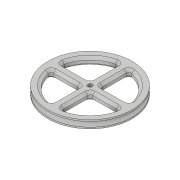
# Autodesk Inventor part: Wheel
Saved by Autodesk Inventor 2017 (Build 210142000, 142)
## iProperties
Created: 2019-06-10
Part Number: Wheel
Material: Generic
Document SubType Name: Modeling
Designer: markg
Density: 1 g/cm^3
Appearance: Default
Author: markg
Autodesk Inventor part; units mm, degrees
ref_plane "YZ Plane" through (0, 0, 0) normal (1, 0, 0) x (0, 1, 0)
ref_plane "XZ Plane" through (0, 0, 0) normal (0, 1, 0) x (-1, 0, 0)
ref_plane "XY Plane" through (0, 0, 0) normal (0, 0, 1) x (1, 0, 0)
sketch "Sketch1" plane through (0, 0, 0) normal (0, 0, 1) x (1, 0, 0)
  line L0 (0, 0) -> (26.9875, 0)
  line L1 (26.9875, 5.08) -> (0, 5.08)
  line L2 (0, 5.08) -> (0, 0)
  arc A0 (26.9875, 4.1275) -> (26.9875, 0.9525) centre (26.9875, 2.54) ccw
  line L3 (26.9875, 0) -> (26.9875, 0.9525)
  line L4 (26.9875, 4.1275) -> (26.9875, 5.08)
  dimension "d0" = 5.08
  dimension "d1" = 26.9875
  dimension "d2" = 3.175
  constraints: 10 end point, 3 parallel, 2 perpendicular, 2 point on circle, 1 centre point, 1 horizontal
  measures "d0" distance of L0.end L1.start
  measures "d1" distance of L1.start L1.end
  measures "d2" diameter of A0
revolve "Revolution1" add sketch "Sketch1" angle 360 about axis through (0, 5.08, 0) along (0, -1, 0)
sketch "Sketch2" plane through (0, 5.08, 0) normal (0, 1, 0) x (1, 0, 0)
  line L0 (-22.0146, 3.0506) -> (-3.175, 3.1571)
  line L1 (3.175, 3.193) -> (21.9787, 3.2993)
  line L2 (-3.175, -21.997) -> (-3.175, -3.193)
  line L3 (-3.175, 3.1571) -> (-3.175, 21.997)
  arc A0 (-3.175, 21.997) -> (-22.0146, 3.0506) centre (0, 0) ccw
  line L4 (-21.9787, -3.2993) -> (-3.175, -3.193)
  line L5 (3.175, -3.1571) -> (22.0146, -3.0506)
  arc A1 (-21.9787, -3.2993) -> (-3.175, -21.997) centre (0, 0) ccw
  line L6 (3.175, -21.997) -> (3.175, -3.1571)
  line L7 (3.175, 3.193) -> (3.175, 21.997)
  arc A2 (3.175, -21.997) -> (22.0146, -3.0506) centre (0, 0) ccw
  arc A3 (21.9787, 3.2993) -> (3.175, 21.997) centre (0, 0) ccw
  constraints: 16 end point, 8 parallel, 8 point on circle, 4 centre point, 2 vertical, 1 coincident
extrude "Extrusion1" cut sketch "Sketch2" against normal blind 25.4
sketch "Sketch3" plane through (0, 5.08, 0) normal (0, 1, 0) x (1, 0, 0)
  arc A0 (-1.0795, -0.9837) -> (-1.0795, 0.9837) centre (0, 0) ccw
  line L0 (-1.0795, -0.9837) -> (-1.0795, 0.9837)
  dimension "d11" = 2.921
  dimension "d12" = 1.0795
  constraints: 2 end point, 2 point on circle, 1 centre point, 1 coincident, 1 vertical
  measures "d11" diameter of A0
  measures "d12" distance from line of L0 point (0, 0)
extrude "Extrusion2" cut sketch "Sketch3" against normal blind 25.4
fillet "Fillet1" radius 1.585 12 edges at (-3.175, 2.54, -3.1571) (3.175, 2.54, -3.193) (3.175, 2.54, 3.1571) (-3.175, 2.54, 3.193) (-21.9787, 2.54, 3.2993) (-3.175, 2.54, 21.997) (3.175, 2.54, 21.997) (22.0146, 2.54, 3.0506) (21.9787, 2.54, -3.2993) (3.175, 2.54, -21.997) (-3.175, 2.54, -21.997) (-22.0146, 2.54, -3.0506)
chamfer "Chamfer1" distance 1.585 angle 45 48 edges at (-12.4262, 5.08, -3.1048) (-21.348, 5.08, -3.6563) (-15.7598, 5.08, -15.671) (-3.7769, 5.08, -21.3269) (-3.175, 5.08, -12.4084) (-3.6361, 5.08, -3.6156) (-12.4172, 5.08, 3.2453) (-3.6424, 5.08, 3.6631) (-3.175, 5.08, 12.4353) (-3.7769, 5.08, 21.3269) (-15.671, 5.08, 15.7598) (-21.3052, 5.08, 3.8974) (12.4262, 5.08, 3.1048) (21.348, 5.08, 3.6563) (15.7598, 5.08, 15.671) (3.7769, 5.08, 21.3269) (3.175, 5.08, 12.4084) (3.6361, 5.08, 3.6156) (12.4172, 5.08, -3.2453) (3.6424, 5.08, -3.6631) (3.175, 5.08, -12.4353) (3.7769, 5.08, -21.3269) (15.671, 5.08, -15.7598) (21.3052, 5.08, -3.8974) (-3.6361, 0, -3.6156) (-12.4262, 0, -3.1048) (-21.348, 0, -3.6563) (-15.7598, 0, -15.671) (-3.7769, 0, -21.3269) (-3.175, 0, -12.4084) (-3.175, 0, 12.4353) (-3.6424, 0, 3.6631) (-12.4172, 0, 3.2453) (-21.3052, 0, 3.8974) (-15.671, 0, 15.7598) (-3.7769, 0, 21.3269) (3.175, 0, 12.4084) (3.7769, 0, 21.3269) (15.7598, 0, 15.671) (21.348, 0, 3.6563) (12.4262, 0, 3.1048) (3.6361, 0, 3.6156) (3.175, 0, -12.4353) (3.6424, 0, -3.6631) (12.4172, 0, -3.2453) (21.3052, 0, -3.8974) (15.671, 0, -15.7598) (3.7769, 0, -21.3269)
body "Solid1"
